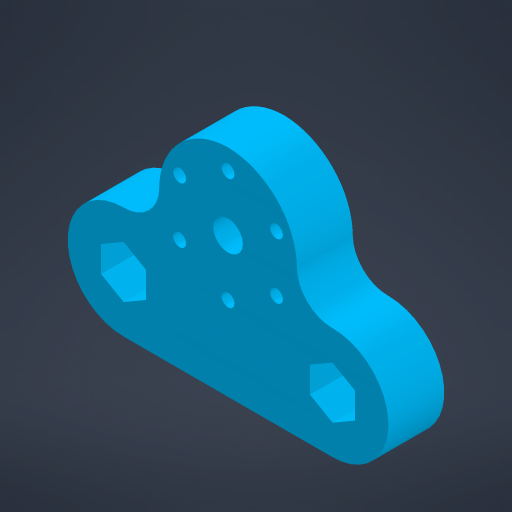
# Autodesk Inventor part: Part2
Saved by Autodesk Inventor 2024.2 (Build 282272000, 272)
## iProperties
Created: 2024-01-12
Part Number: Part2
Material: Generic
Document SubType Name: Modeling
Designer: AdminForWorker
Density: 1 g/cm^3
Appearance: Default
Author: AdminForWorker
Autodesk Inventor part; units mm, degrees
ref_plane "YZ Plane" through (0, 0, 0) normal (1, 0, 0) x (0, 1, 0)
ref_plane "XZ Plane" through (0, 0, 0) normal (0, 1, 0) x (-1, 0, 0)
ref_plane "XY Plane" through (0, 0, 0) normal (0, 0, 1) x (1, 0, 0)
sketch "Sketch7" plane through (0, 0, 0) normal (0, 0, 1) x (1, 0, 0)
  line L0 (64.7605, 16) -> (64.8102, 16)
  circle A0 centre (34.904, 8) radius 1.85
  line L1 (34.904, 0) -> (21.0475, 0)
  circle A1 centre (21.0475, 32) radius 1.85
  circle A2 centre (48.7605, 32) radius 1.85
  circle A3 centre (48.7605, 16) radius 1.85
  circle A4 centre (21.0475, 16) radius 1.85
  line L2 (34.904, -16) -> (33.054, -16)
  line L3 (4.9978, -16) -> (29.0539, -16)
  line L4 (44.974, -16) -> (64.8102, -16)
  circle A5 centre (34.904, 40) radius 1.85
  line L5 (4.9978, 16) -> (5.1975, 16)
  line L6 (64.6105, 16) -> (64.8102, 16)
  line L7 (34.904, 8) -> (34.904, 24)
  circle A6 centre (34.904, 24) radius 4.25
  line L8 (29.0539, -16) -> (44.974, -16)
  line L9 (34.904, 40) -> (34.904, 41.85)
  line L10 (34.904, 41.85) -> (34.904, 45.85)
  line L11 (21.0475, 16) -> (19.1975, 16)
  line L12 (19.1975, 16) -> (15.1975, 16)
  line L13 (48.7605, 16) -> (50.6105, 16)
  line L14 (15.1975, 26) -> (15.1975, 25.85)
  line L15 (35.1975, 45.85) -> (34.904, 45.85)
  line L16 (54.6105, 26) -> (54.6105, 25.85)
  line L17 (34.6105, 45.85) -> (34.904, 45.85)
  arc A7 (35.1975, 45.85) -> (15.1975, 25.85) centre (35.1975, 25.85) ccw
  arc A8 (54.6105, 25.85) -> (34.6105, 45.85) centre (34.6105, 25.85) ccw
  arc A9 (5.1975, 16) -> (15.1975, 26) centre (5.1975, 26) ccw
  arc A10 (54.6105, 26) -> (64.6105, 16) centre (64.6105, 26) ccw
  line L18 (48.8102, 0) -> (58.36, 0)
  line L19 (58.36, 0) -> (48.8102, 0)
  line L20 (11.448, 3.724) -> (11.448, -3.724)
  line L21 (11.448, 3.724) -> (18.896, 3.724) construction
  line L22 (11.448, 3.724) -> (18.896, 3.724) construction
  line L23 (11.448, -3.724) -> (6.2803, -6.7076)
  line L24 (11.448, -3.724) -> (17.4152, -3.724) construction
  line L25 (11.448, -3.724) -> (4.9978, -7.448)
  line L26 (4.9978, -7.448) -> (-1.4523, -3.724)
  line L27 (-1.4523, -3.724) -> (-1.4523, 3.724)
  line L28 (-1.4523, 3.724) -> (4.9978, 7.448)
  line L29 (4.9978, 7.448) -> (11.448, 3.724)
  line L30 (11.448, 0) -> (48.8102, 0)
  line L31 (58.36, 3.724) -> (58.36, -3.724)
  line L32 (58.36, 3.724) -> (50.912, 3.724) construction
  line L33 (58.36, 3.724) -> (50.912, 3.724) construction
  line L34 (58.36, -3.724) -> (63.5277, -6.7076)
  line L35 (58.36, -3.724) -> (52.3928, -3.724) construction
  line L36 (58.36, -3.724) -> (64.8102, -7.448)
  line L37 (64.8102, -7.448) -> (71.2603, -3.724)
  line L38 (71.2603, -3.724) -> (71.2603, 3.724)
  line L39 (71.2603, 3.724) -> (64.8102, 7.448)
  line L40 (64.8102, 7.448) -> (58.36, 3.724)
  line L41 (4.9978, 7.448) -> (4.9978, 0)
  arc A11 (4.9978, 16) -> (4.9978, -16) centre (4.9978, 0) ccw
  line L42 (64.8102, 7.448) -> (64.8102, 0)
  arc A12 (48.8102, 0) -> (64.8102, 16) centre (64.8102, 0) ccw
  point P0 (54.6105, 45.85)
  point P1 (34.904, 45.8479)
  point P2 (34.904, 45.8479)
  point P3 (69.808, 16)
  point P4 (11.448, 0)
  point P5 (34.904, 45.8479)
  point P6 (58.36, 0)
  dimension "d83" = 16
  dimension "d84" = 8.5
  dimension "d85" = 4
  dimension "d86" = 4
  dimension "d88" = 20
  dimension "d89" = 10
  dimension "d93" = 23.456
  dimension "d94" = 46.912
  dimension "d96" = 7.448
  dimension "d105" = 150
  dimension "d106" = 7.448
  dimension "d107" = 7.448
  dimension "d108" = 120
  dimension "d109" = 7.448
  dimension "d110" = 7.448
  dimension "d111" = 32
  dimension "d112" = 32
  constraints: 86 end point, 13 point on circle, 12 symmetric about line, 10 centre point, 10 point on line, 8 tangent, 6 horizontal, 6 vertical, 3 coincident, 3 perpendicular, 2 equal radius, 2 horizontal alignment, 2 parallel, 1 collinear, 1 equal length, 1 vertical alignment, 6 other
  measures "d83" distance of L7.start L7.end
  measures "d84" diameter of A6
  measures "d85" distance of L9.end L10.end
  measures "d86" distance of L11.end L12.end
  measures "d88" radius of A7
  measures "d89" radius of A9
  measures "d93" distance of L1.start L18.end
  measures "d94" distance of L18.end point (11.448, 0)
  measures "d96" distance of L20.start L20.end
  measures "d105" angle of L23 L24
  measures "d106" distance of L20.end L25.end
  measures "d107" distance of L25.end L26.end
  measures "d108" angle of L25 L26
  measures "d109" distance of L26.end L27.end
  measures "d110" distance of L27.end L28.end
  measures "d111" diameter of A11
  measures "d112" diameter of A12
extrude "Extrusion3" add sketch "Sketch7" along normal blind 16
body "Solid4"
